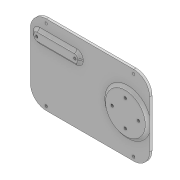
# Autodesk Inventor part: base_barra_bola
Saved by Autodesk Inventor 2022 (Build 260153000, 153)
## iProperties
Created: 2022-11-06
Part Number: base_barra_bola
Material: Genérico
Document SubType Name: Modeling
Designer: Jorge
Density: 1 g/cm^3
Appearance: Valor por defecto
Author: Jorge
Autodesk Inventor part; units mm, degrees
ref_plane "YZ Plane" through (0, 0, 0) normal (1, 0, 0) x (0, 1, 0)
ref_plane "XZ Plane" through (0, 0, 0) normal (0, 1, 0) x (-1, 0, 0)
ref_plane "XY Plane" through (0, 0, 0) normal (0, 0, 1) x (1, 0, 0)
sketch "Boceto1" plane through (0, 0, 0) normal (0, 0, 1) x (1, 0, 0)
  line L0 (0, 0) -> (150, 0)
  line L1 (150, 0) -> (150, 100)
  line L2 (150, 100) -> (0, 100)
  line L3 (0, 100) -> (0, 0)
  dimension "d0" = 150
  dimension "d1" = 100
  constraints: 8 end point, 2 parallel, 1 horizontal, 1 perpendicular
  measures "d0" distance of L2.end L1.end
  measures "d1" distance of L1.end L0.end
extrude "Extrusión1" add sketch "Boceto1" along normal blind 3
sketch "Boceto2" plane through (0, 0, 3) normal (0, 0, 1) x (1, 0, 0)
  line L0 (150, 0) -> (150, 100) construction
  line L1 (150, 100) -> (0, 100) construction
  line L2 (0, 100) -> (0, 0) construction
  line L3 (0, 0) -> (150, 0) construction
  line L4 (0, 100) -> (0, 0) construction
  line L5 (0, 50) -> (150, 50) construction
  line L6 (150, 0) -> (150, 100) construction
  line L7 (150, 100) -> (0, 100) construction
  line L8 (122.5, 100) -> (122.5, 0) construction
  line L9 (0, 0) -> (150, 0) construction
  line L10 (0, 66.5) -> (150, 66.5) construction
  line L11 (0, 33.5) -> (150, 33.5) construction
  line L12 (106, 100) -> (106, 0) construction
  line L13 (139, 100) -> (139, 0) construction
  circle A0 centre (106, 50) radius 1.1
  circle A1 centre (122.5, 66.5) radius 1.1
  circle A2 centre (139, 50) radius 1.1
  circle A3 centre (122.5, 33.5) radius 1.1
  line L14 (0, 77.8) -> (150, 77.8) construction
  line L15 (35, 100) -> (35, 0) construction
  line L16 (11, 100) -> (11, 0) construction
  line L17 (59, 100) -> (59, 0) construction
  circle A4 centre (11, 77.8) radius 1.1
  circle A5 centre (59, 77.8) radius 1.1
  line L18 (75, 100) -> (75, 0) construction
  dimension "d4" = 33
  dimension "d5" = 16.5
  dimension "d6" = 33
  dimension "d7" = 16.5
  dimension "d8" = 2.2
  dimension "d9" = 2.2
  dimension "d10" = 2.2
  dimension "d11" = 2.2
  dimension "d15" = 48
  dimension "d16" = 24
  dimension "d17" = 47
  dimension "d18" = 27.8
  dimension "d19" = 2.2
  dimension "d20" = 2.2
  dimension "d22" = 128
  dimension "d24" = 64
  constraints: 22 end point, 14 point on line, 7 perpendicular, 6 centre point, 4 midpoint, 2 vertical, 16 other
  measures "d4" distance between parallel lines of L13 L12
  measures "d5" distance between parallel lines of L8 L12
  measures "d6" distance between parallel lines of L11 L10
  measures "d7" distance between parallel lines of L5 L10
  measures "d8" diameter of A0
  measures "d9" diameter of A1
  measures "d10" diameter of A2
  measures "d11" diameter of A3
  measures "d15" distance between parallel lines of L17 L16
  measures "d16" distance between parallel lines of L15 L16
  measures "d17" distance between parallel lines of L17 L12
  measures "d18" distance between parallel lines of L5 L14
  measures "d19" diameter of A4
  measures "d20" diameter of A5
  measures "d22" distance between parallel lines of L13 L16
  measures "d24" distance between parallel lines of L18 L16
extrude "Extrusión2" cut sketch "Boceto2" against normal blind 10
fillet "Empalme1" radius 20 4 edges at (150, 0, 1.5) (150, 100, 1.5) (0, 100, 1.5) (0, 0, 1.5)
sketch "Boceto3" plane through (0, 0, 3) normal (0, 0, 1) x (1, 0, 0)
  circle A0 centre (122.5, 33.5) radius 1.1 construction
  circle A1 centre (106, 50) radius 1.1 construction
  circle A2 centre (11, 77.8) radius 1.1 construction
  circle A3 centre (122.5, 66.5) radius 1.1 construction
  circle A4 centre (139, 50) radius 1.1 construction
  circle A5 centre (59, 77.8) radius 1.1 construction
  arc A6 (0, 20) -> (20, 0) centre (20, 20) ccw construction
  line L0 (20, 0) -> (130, 0) construction
  arc A7 (130, 0) -> (150, 20) centre (130, 20) ccw construction
  line L1 (150, 20) -> (150, 80) construction
  arc A8 (150, 80) -> (130, 100) centre (130, 80) ccw construction
  line L2 (130, 100) -> (20, 100) construction
  arc A9 (20, 100) -> (0, 80) centre (20, 80) ccw construction
  line L3 (0, 80) -> (0, 20) construction
  circle A10 centre (122.5, 66.5) radius 1.1 construction
  line L4 (122.5, 66.5) -> (122.5, 33.5) construction
  circle A11 centre (122.5, 50) radius 25
  line L5 (7.5, 82.8) -> (62.5, 82.8)
  line L6 (62.5, 82.8) -> (62.5, 72.8)
  line L7 (62.5, 72.8) -> (7.5, 72.8)
  line L8 (7.5, 72.8) -> (7.5, 82.8)
  circle A12 centre (11, 77.8) radius 1.1 construction
  circle A13 centre (59, 77.8) radius 1.1 construction
  line L9 (11, 77.8) -> (59, 77.8) construction
  point P0 (0, 0)
  point P1 (35, 77.8)
  dimension "d25" = 50
  dimension "d26" = 10
  dimension "d27" = 55
  dimension "d28" = 27.5
  dimension "d29" = 5
  constraints: 12 end point, 2 horizontal, 2 midpoint, 2 parallel, 1 centre point, 1 perpendicular, 1 vertical
  measures "d25" diameter of A11
  measures "d26" distance between parallel lines of L7 L5
  measures "d27" distance between parallel lines of L6 L8
  measures "d28" distance from line of point (35, 77.8) L8
  measures "d29" distance between parallel lines of L7 L9
extrude "Extrusión3" add sketch "Boceto3" along normal blind 3
fillet "Empalme2" radius 4 4 edges at (62.5, 82.8, 4.5) (7.5, 82.8, 4.5) (62.5, 72.8, 4.5) (7.5, 72.8, 4.5)
fillet "Empalme3" radius 4 9 edges at (8.6716, 73.9716, 3) (7.5, 77.8, 3) (8.6716, 81.6284, 3) (35, 82.8, 3) (61.3284, 81.6284, 3) (62.5, 77.8, 3) (61.3284, 73.9716, 3) (35, 72.8, 3) (97.5, 50, 3)
sketch "Boceto4" plane through (0, 0, 0) normal (0, 0, -1) x (-1, 0, 0)
  arc A0 (-20, 0) -> (0, 20) centre (-20, 20) ccw construction
  line L0 (0, 80) -> (0, 20) construction
  arc A1 (0, 80) -> (-20, 100) centre (-20, 80) ccw construction
  line L1 (-130, 100) -> (-20, 100) construction
  arc A2 (-130, 100) -> (-150, 80) centre (-130, 80) ccw construction
  line L2 (-150, 20) -> (-150, 80) construction
  arc A3 (-150, 20) -> (-130, 0) centre (-130, 20) ccw construction
  line L3 (-20, 0) -> (-130, 0) construction
  circle A4 centre (-122.5, 33.5) radius 1.1 construction
  circle A5 centre (-106, 50) radius 1.1 construction
  circle A6 centre (-11, 77.8) radius 1.1 construction
  circle A7 centre (-122.5, 66.5) radius 1.1 construction
  circle A8 centre (-139, 50) radius 1.1 construction
  circle A9 centre (-59, 77.8) radius 1.1 construction
  circle A10 centre (-122.5, 33.5) radius 1.1 projected
  circle A11 centre (-122.5, 33.5) radius 1.9
  circle A12 centre (-106, 50) radius 1.1 projected
  circle A13 centre (-106, 50) radius 1.9
  circle A14 centre (-139, 50) radius 1.1 projected
  circle A15 centre (-139, 50) radius 1.9
  circle A16 centre (-122.5, 66.5) radius 1.1 projected
  circle A17 centre (-122.5, 66.5) radius 1.9
  circle A18 centre (-11, 77.8) radius 1.1 projected
  circle A19 centre (-11, 77.8) radius 1.9
  circle A20 centre (-59, 77.8) radius 1.1 projected
  circle A21 centre (-59, 77.8) radius 1.9
  point P0 (0, 0)
  dimension "d34" = 3.8
  dimension "d35" = 3.8
  dimension "d36" = 3.8
  dimension "d37" = 3.8
  dimension "d38" = 3.8
  dimension "d39" = 3.8
  constraints: 6 centre point, 6 coincident
  measures "d34" diameter of A11
  measures "d35" diameter of A13
  measures "d36" diameter of A15
  measures "d37" diameter of A17
  measures "d38" diameter of A19
  measures "d39" diameter of A21
extrude "Extrusión4" cut sketch "Boceto4" against normal blind 5 contours A10 | A11 | A12 | A13 | A14 | A15 | A16 | A17 | A18 | A19 | A20 | A21
sketch "Boceto5" plane through (122.5, 33.5, 5) normal (0, 0, -1) x (-1, 0, 0)
  circle A0 centre (111.5, 44.3) radius 1.9 construction
  circle A1 centre (0, 0) radius 1.9 construction
  circle A2 centre (16.5, 16.5) radius 1.9 construction
  circle A3 centre (63.5, 44.3) radius 1.9 construction
  circle A4 centre (0, 33) radius 1.9 construction
  circle A5 centre (-16.5, 16.5) radius 1.9 construction
  arc A6 (102.5, -33.5) -> (122.5, -13.5) centre (102.5, -13.5) ccw construction
  line L0 (122.5, 46.5) -> (122.5, -13.5) construction
  arc A7 (122.5, 46.5) -> (102.5, 66.5) centre (102.5, 46.5) ccw construction
  line L1 (-7.5, 66.5) -> (102.5, 66.5) construction
  arc A8 (-7.5, 66.5) -> (-27.5, 46.5) centre (-7.5, 46.5) ccw construction
  line L2 (-27.5, -13.5) -> (-27.5, 46.5) construction
  arc A9 (-27.5, -13.5) -> (-7.5, -33.5) centre (-7.5, -13.5) ccw construction
  line L3 (102.5, -33.5) -> (-7.5, -33.5) construction
  circle A10 centre (0, 0) radius 1.9 projected
  circle A11 centre (0, 0) radius 1.6
  circle A12 centre (16.5, 16.5) radius 1.9 projected
  circle A13 centre (16.5, 16.5) radius 1.6
  circle A14 centre (-16.5, 16.5) radius 1.9 projected
  circle A15 centre (-16.5, 16.5) radius 1.6
  circle A16 centre (0, 33) radius 1.9 projected
  circle A17 centre (0, 33) radius 1.6
  circle A18 centre (63.5, 44.3) radius 1.9 projected
  circle A19 centre (63.5, 44.3) radius 1.6
  circle A20 centre (111.5, 44.3) radius 1.9 projected
  circle A21 centre (111.5, 44.3) radius 1.6
  point P0 (122.5, -33.5)
  dimension "d42" = 3.2
  dimension "d43" = 3.2
  dimension "d44" = 3.2
  dimension "d45" = 3.2
  dimension "d46" = 3.2
  dimension "d47" = 3.2
  constraints: 6 centre point, 6 coincident
  measures "d42" diameter of A11
  measures "d43" diameter of A13
  measures "d44" diameter of A15
  measures "d45" diameter of A17
  measures "d46" diameter of A19
  measures "d47" diameter of A21
extrude "Extrusión5" cut sketch "Boceto5" against normal through all contours A11 | A13 | A15 | A17 | A19 | A21
sketch "Boceto6" plane through (0, 0, 3) normal (0, 0, 1) x (1, 0, 0)
  arc A0 (150, 58.7977) -> (150, 41.2023) centre (122.5, 50) ccw construction
  line L0 (150, 58.7977) -> (150, 80) construction
  arc A1 (150, 80) -> (130, 100) centre (130, 80) ccw construction
  line L1 (130, 100) -> (20, 100) construction
  arc A2 (20, 100) -> (0, 80) centre (20, 80) ccw construction
  line L2 (0, 80) -> (0, 20) construction
  arc A3 (0, 20) -> (20, 0) centre (20, 20) ccw construction
  line L3 (20, 0) -> (130, 0) construction
  arc A4 (130, 0) -> (150, 20) centre (130, 20) ccw construction
  line L4 (150, 20) -> (150, 41.2023) construction
  line L5 (11.5, 68.927) -> (58.5, 68.927) construction
  arc A5 (3.627, 76.8) -> (11.5, 68.927) centre (11.5, 76.8) ccw construction
  line L6 (3.627, 78.8) -> (3.627, 76.8) construction
  arc A6 (11.5, 86.673) -> (3.627, 78.8) centre (11.5, 78.8) ccw construction
  line L7 (58.5, 86.673) -> (11.5, 86.673) construction
  arc A7 (66.373, 78.8) -> (58.5, 86.673) centre (58.5, 78.8) ccw construction
  line L8 (66.373, 76.8) -> (66.373, 78.8) construction
  arc A8 (58.5, 68.927) -> (66.373, 76.8) centre (58.5, 76.8) ccw construction
  line L9 (0, 80) -> (0, 20) construction
  line L10 (0, 95) -> (150, 95) construction
  line L11 (150, 58.7977) -> (150, 80) construction
  line L12 (0, 5) -> (150, 5) construction
  line L13 (150, 20) -> (150, 80) construction
  line L14 (130, 100) -> (20, 100) construction
  line L15 (20, 100) -> (20, 0) construction
  line L16 (20, 0) -> (130, 0) construction
  line L17 (130, 100) -> (130, 0) construction
  circle A9 centre (20, 95) radius 1.6
  circle A10 centre (130, 95) radius 1.6
  circle A11 centre (20, 5) radius 1.6
  circle A12 centre (130, 5) radius 1.6
  point P0 (0, 0)
  dimension "d50" = 20
  dimension "d51" = 5
  dimension "d52" = 20
  dimension "d53" = 5
  dimension "d54" = 3.2
  dimension "d55" = 3.2
  dimension "d56" = 3.2
  dimension "d57" = 3.2
  constraints: 16 point on line, 8 end point, 4 centre point, 4 perpendicular
  measures "d50" distance between parallel lines of L2 L15
  measures "d51" distance between parallel lines of L1 L10
  measures "d52" distance between parallel lines of L0 L17
  measures "d53" distance between parallel lines of L3 L12
  measures "d54" diameter of A9
  measures "d55" diameter of A10
  measures "d56" diameter of A11
  measures "d57" diameter of A12
extrude "Extrusión6" cut sketch "Boceto6" against normal through all
equation "\"d5\" = 0.5 * d4"
equation "\"d7\" = d5"
equation "\"d16\" = 0.5 * d15"
equation "\"d24\" = 0.5 * d22"
equation "\"d28\" = 0.5 * d27"
equation "\"d29\" = 0.5 * d26"
